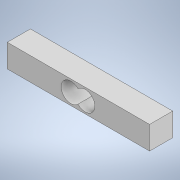
# Autodesk Inventor part: Weight_Sensor
Saved by Autodesk Inventor 2021 (Build 250183000, 183)
## iProperties
Created: 2022-02-21
Part Number: Weight_Sensor
Material: Generic
Document SubType Name: Modeling
Designer: aerts
Density: 1 g/cm^3
Appearance: Default
Author: aerts
Autodesk Inventor part; units mm, degrees
ref_plane "YZ Plane" through (0, 0, 0) normal (1, 0, 0) x (0, 1, 0)
ref_plane "XZ Plane" through (0, 0, 0) normal (0, 1, 0) x (-1, 0, 0)
ref_plane "XY Plane" through (0, 0, 0) normal (0, 0, 1) x (1, 0, 0)
sketch "Sketch1" plane through (0, 0, 0) normal (0, 0, 1) x (1, 0, 0)
  line L0 (0, 0) -> (80, 0)
  line L1 (80, 0) -> (80, 13)
  line L2 (80, 13) -> (0, 13)
  line L3 (0, 13) -> (0, 0)
  dimension "d0" = 80
  dimension "d1" = 13
  constraints: 8 end point, 2 parallel, 1 horizontal, 1 perpendicular
  measures "d0" distance of L1.end L2.end
  measures "d1" distance of L0.end L1.end
extrude "Extrusion1" add sketch "Sketch1" along normal blind 13
sketch "Sketch2" plane through (0, 0, 13) normal (0, 0, 1) x (1, 0, 0)
  circle A0 centre (35.7535, 6.5) radius 5.5
  circle A1 centre (43.7535, 6.4786) radius 5.5
  line L0 (80, 13) -> (0, 13) projected
  line L1 (80, 0) -> (80, 13) projected
  line L2 (0, 13) -> (0, 0) projected
  line L3 (80, 0) -> (80, 13) projected
  line L4 (80, 13) -> (0, 13) projected
  line L5 (0, 13) -> (0, 0) projected
  line L6 (0, 0) -> (80, 0) projected
  point P0 (39.7636, 10.2642)
  point P1 (39.7434, 2.7144)
  point P2 (40, 13)
  dimension "d14" = 13
  dimension "d15" = 80
  dimension "d17" = 40
  dimension "d18" = 19
  dimension "d19" = 6.5
  dimension "d20" = 8
  constraints: 2 centre point, 1 midpoint
  measures "d14" distance of L0.end L2.end
  measures "d15" distance of L5.end L3.start
  measures "d17" distance from line of L1 point (40, 13)
  measures "d19" distance from line of L0 A0.centre
  measures "d20" horizontal distance of A1.centre A0.centre
extrude "Extrusion2" cut sketch "Sketch2" against normal blind 13 contours A0 A1 | A0 A1 | A1 A0
body "Solid1"
